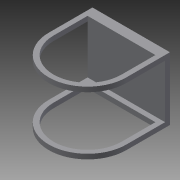
# Autodesk Inventor part: router_mount
Saved by Autodesk Inventor 2014 (Build 180170000, 170)
## iProperties
Created: 2014-08-20
Part Number: router_mount
Material: Generic
Document SubType Name: Modeling
Designer: Matthew
Density: 1 g/cm^3
Appearance: Default
Author: Matthew
Autodesk Inventor part; units mm, degrees
ref_plane "YZ Plane" through (0, 0, 0) normal (1, 0, 0) x (0, 1, 0)
ref_plane "XZ Plane" through (0, 0, 0) normal (0, 1, 0) x (-1, 0, 0)
ref_plane "XY Plane" through (0, 0, 0) normal (0, 0, 1) x (1, 0, 0)
sketch "Sketch1" plane through (0, 0, 0) normal (0, 1, 0) x (-1, 0, 0)
  line L0 (50.8, -50.8) -> (-50.8, -50.8)
  line L1 (50.8, -50.8) -> (50.8, 0)
  line L2 (-50.8, -50.8) -> (-50.8, 0)
  arc A0 (50.8, 0) -> (-50.8, 0) centre (0, 0) ccw
  line L3 (44.45, -44.45) -> (-44.45, -44.45)
  line L4 (-44.45, -44.45) -> (-44.45, 0)
  line L5 (44.45, -44.45) -> (44.45, 0)
  arc A1 (44.45, 0) -> (-44.45, 0) centre (0, 0) ccw
  dimension "d2" = 101.6
  dimension "d4" = 6.35
  dimension "d5" = 6.35
  dimension "d6" = 6.35
  dimension "d34" = 44.45
  dimension "d36" = 44.45
  constraints: 12 end point, 4 point on circle, 4 tangent, 3 perpendicular, 2 centre point, 2 coincident, 2 parallel, 2 vertical alignment, 1 horizontal
  measures "d2" distance of L0.start L0.end
  measures "d4" distance between parallel lines of L0 L3
  measures "d5" distance between parallel lines of L2 L4
  measures "d6" distance between parallel lines of L1 L5
  measures "d34" radius of A1
  measures "d36" distance of L3.end L4.end
extrude "Extrusion1" add sketch "Sketch1" along normal blind 6.35
sketch "Sketch2" plane through (50.8, 0, -50.8) normal (0, 0, -1) x (-1, 0, 0)
  line L0 (101.6, 0) -> (101.6, 6.35) projected
  line L1 (0, 6.35) -> (101.6, 6.35) projected
  line L2 (0, 0) -> (0, 6.35) projected
  point P0 (50.8, 0)
  point P1 (3.175, 3.175)
  point P2 (98.425, 3.175)
  dimension "d9" = 3.175
  dimension "d10" = 3.175
  dimension "d11" = 3.175
  constraints: 1 horizontal alignment
  measures "d9" distance from line of L2 point (3.175, 3.175)
  measures "d10" distance from line of L0 point (98.425, 3.175)
  measures "d11" distance from line of L1 point (3.175, 3.175)
hole "Hole1" at (47.625, 3.175, -50.8) at (-47.625, 3.175, -50.8) direction (0, 0, 1) diameter 4.826 depth 25.4
pattern_linear "Rectangular Pattern1" count 2 spacing 76.2 along (0, 1, 0) of "Extrusion1"
sketch "Sketch3" plane through (50.8, 76.2, -50.8) normal (0, 0, -1) x (-1, 0, 0)
  line L0 (101.6, 0) -> (101.6, 6.35) projected
  line L1 (0, 6.35) -> (101.6, 6.35) projected
  line L2 (0, 0) -> (0, 6.35) projected
  point P0 (50.8, -76.2)
  point P1 (3.175, 3.175)
  point P2 (98.425, 3.175)
  dimension "d22" = 3.175
  dimension "d23" = 3.175
  dimension "d24" = 3.175
  constraints: 1 horizontal alignment
  measures "d22" distance from line of L2 point (3.175, 3.175)
  measures "d23" distance from line of L0 point (98.425, 3.175)
  measures "d24" distance from line of L1 point (3.175, 3.175)
hole "Hole2" at (47.625, 79.375, -50.8) at (-47.625, 79.375, -50.8) direction (0, 0, 1) diameter 4.826 depth 25.4
sketch "Sketch4" plane through (50.8, 76.2, -50.8) normal (0, 0, -1) x (-1, 0, 0)
  circle A0 centre (3.175, 3.175) radius 2.413 projected
  circle A1 centre (98.425, 3.175) radius 2.413 projected
  line L0 (101.6, 0) -> (0, 0) construction
  line L1 (0, 6.35) -> (101.6, 6.35) projected
  line L2 (0, 0) -> (0, 6.35) projected
  line L3 (0, 6.35) -> (0, -76.2)
  line L4 (0, -76.2) -> (101.6, -76.2)
  line L5 (101.6, -76.2) -> (101.6, 6.35)
  line L6 (0, 6.35) -> (101.6, 6.35)
  point P0 (50.8, -76.2)
  constraints: 10 end point, 2 collinear, 1 parallel, 1 perpendicular
extrude "Extrusion2" add sketch "Sketch4" along normal blind 6.35
equation "\"d5\" = d4"
equation "\"d6\" = d4"
equation "\"d10\" = d9"
equation "\"d23\" = d22"
body "Solid1"
